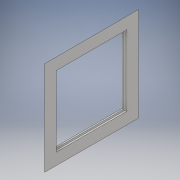
# Autodesk Inventor part: PV_Rahmen
Saved by Autodesk Inventor 2018.3 (Build 223284000, 284)
## iProperties
Created: 2019-11-04
Part Number: PV_Rahmen
Material: Generisch
Document SubType Name: Modeling
Designer: DerLobre
Density: 1 g/cm^3
Appearance: Vorgabe
Author: DerLobre
Autodesk Inventor part; units mm, degrees
ref_plane "YZ Plane" through (0, 0, 0) normal (1, 0, 0) x (0, 1, 0)
ref_plane "XZ Plane" through (0, 0, 0) normal (0, 1, 0) x (-1, 0, 0)
ref_plane "XY Plane" through (0, 0, 0) normal (0, 0, 1) x (1, 0, 0)
sketch "Skizze1" plane through (0, 0, 0) normal (1, 0, 0) x (0, 1, 0)
  line L0 (-270, 270) -> (270, 270)
  line L1 (270, 270) -> (270, -270)
  line L2 (270, -270) -> (-270, -270)
  line L3 (-270, -270) -> (-270, 270)
  line L4 (-378, 0) -> (378, 0) projected
  line L5 (0, -378) -> (0, 378) projected
  point P0 (0, 0)
  dimension "d0" = 540
  dimension "d1" = 540
  constraints: 8 end point, 2 parallel, 1 horizontal, 1 perpendicular, 2 other
  measures "d0" distance of L0.start L0.end
  measures "d1" distance of L2.end L0.start
extrude "Extrusion1" add sketch "Skizze1" along normal blind 18
sketch "Skizze2" plane through (18, 0, 0) normal (1, 0, 0) x (0, 0, -1)
  line L0 (-270, 270) -> (-270, -270) projected
  line L1 (-270, -270) -> (270, -270) projected
  line L2 (270, -270) -> (270, 270) projected
  line L3 (270, 270) -> (-270, 270) projected
  line L4 (-203, -203) -> (203, -203)
  line L5 (203, -203) -> (203, 203)
  line L6 (203, 203) -> (-203, 203)
  line L7 (-203, 203) -> (-203, -203)
  point P0 (0, 0)
  dimension "d4" = 67
  dimension "d5" = 67
  dimension "d6" = 67
  dimension "d7" = 67
  constraints: 8 end point, 2 parallel, 1 horizontal, 1 perpendicular
  measures "d4" distance between parallel lines of L2 L5
  measures "d5" distance between parallel lines of L3 L6
  measures "d6" distance between parallel lines of L0 L7
  measures "d7" distance between parallel lines of L1 L4
extrude "Extrusion2" cut sketch "Skizze2" against normal blind 10 contours L7 L6 L5 L4
sketch "Skizze3" plane through (8, 0, 0) normal (1, 0, 0) x (0, 0, -1)
  line L0 (203, -203) -> (-203, -203) projected
  line L1 (203, 203) -> (203, -203) projected
  line L2 (-203, 203) -> (203, 203) projected
  line L3 (-203, -203) -> (-203, 203) projected
  line L4 (-193, -193) -> (193, -193)
  line L5 (193, -193) -> (193, 193)
  line L6 (193, 193) -> (-193, 193)
  line L7 (-193, 193) -> (-193, -193)
  point P0 (0, 0)
  dimension "d10" = 10
  dimension "d11" = 10
  dimension "d12" = 10
  dimension "d13" = 10
  constraints: 8 end point, 2 parallel, 1 horizontal, 1 perpendicular
  measures "d10" distance between parallel lines of L1 L5
  measures "d11" distance between parallel lines of L2 L6
  measures "d12" distance between parallel lines of L3 L7
  measures "d13" distance between parallel lines of L0 L4
extrude "Extrusion3" cut sketch "Skizze3" against normal blind 8 contours L7 L6 L5 L4
sketch "Skizze6" plane through (0, 0, 0) normal (-1, 0, 0) x (0, 0, 1)
  line L0 (-193, -193) -> (-193, 193) projected
  line L1 (-193, 193) -> (193, 193) projected
  line L2 (193, 193) -> (193, -193) projected
  line L3 (193, -193) -> (-193, -193) projected
  line L4 (270, -270) -> (270, 270) projected
  line L5 (270, 270) -> (-270, 270) projected
  line L6 (-270, 270) -> (-270, -270) projected
  line L7 (-270, -270) -> (270, -270) projected
  line L8 (17.5, -201) -> (17.5, -210) projected
  line L9 (22, -201) -> (17.5, -201) projected
  line L10 (17.5, -210) -> (13, -210) projected
  line L11 (13, -197) -> (13, -210) projected
  line L12 (22, -197) -> (22, -201) projected
  line L13 (-200, -197) -> (200, -197) projected
  line L14 (11, -197) -> (11, -210) projected
  line L15 (2, -197) -> (2, -201) projected
  line L16 (6.5, -201) -> (2, -201) projected
  line L17 (6.5, -201) -> (6.5, -210) projected
  line L18 (11, -210) -> (6.5, -210) projected
  line L19 (-5, -197) -> (-5, -201) projected
  line L20 (-5, -201) -> (-9.5, -201) projected
  line L21 (-9.5, -201) -> (-9.5, -210) projected
  line L22 (-9.5, -210) -> (-14, -210) projected
  line L23 (-14, -197) -> (-14, -210) projected
  line L24 (-16, -197) -> (-16, -210) projected
  line L25 (-16, -210) -> (-20.5, -210) projected
  line L26 (-20.5, -201) -> (-20.5, -210) projected
  line L27 (-20.5, -201) -> (-25, -201) projected
  line L28 (-25, -197) -> (-25, -201) projected
  line L29 (-270, -270) -> (270, -270) projected
  line L30 (-25, -243) -> (-25, -193)
  line L31 (25, -243) -> (25, -193)
  line L32 (0, -378) -> (0, 378) projected
  line L33 (-378, 0) -> (378, 0) projected
  line L34 (25, -243) -> (-25, -243)
  line L35 (25, -193) -> (-25, -193)
  point P0 (0, 0)
  dimension "d34" = 50
  dimension "d37" = 50
  constraints: 8 end point, 3 perpendicular, 2 point on line, 1 collinear, 2 other
  measures "d34" distance between parallel lines of L30 L31
  measures "d37" distance between parallel lines of L34 L3
chamfer "Fase1" distance 18 angle 45 1 edges at (0, -270, 0)
chamfer "Fase2" distance 18 angle 45 2 edges at (0, 270, 0) (0, 8.9999, 270)
extrude "Extrusion7" cut sketch "Skizze6" against normal blind 15 contours L0 L33 L32 L3 | L0 L1 L32 L33 | L3 L32 L13 L30 | L33 L2 L3 L32 | L32 L1 L2 L33 | L3 L31 L13 L32 | L13 L24 L25 L26 L27 L28 | L32 L34 L30 L27 L26 L25 L24 L13 L23 L22 L21 L20 L19 | L13 L15 L16 L17 L18 L14 L11 L10 L8 L9 L12 L31 L34 L32 | L19 L20 L21 L22 L23 L13 | L13 L14 L18 L17 L16 L15 | L12 L9 L8 L10 L11 L13
